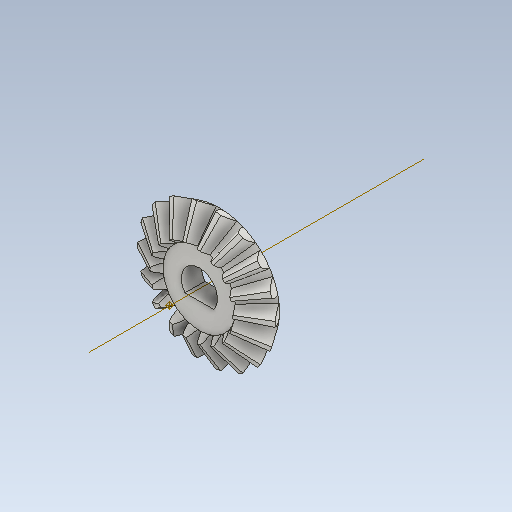
# Autodesk Inventor part: Коническая зубчатая передача2
Saved by Autodesk Inventor 2020 (Build 240168000, 168)
## iProperties
Created: 2021-02-28
Part Number: Коническая зубчатая передача2
Material: Steel, Mild
Document SubType Name: Modeling
Designer: Антон
Categories: <?xml version="1.0" encoding="UTF-16"?> <MemberInstance><Categories><FamilyTemplate><FamilyTemplateParameter ValueType="xs:double" Id="1" ObjectReferenceKey="da_z" ObjectType="kUserParameterObject"/><FamilyTemplateParameter ValueType="xs:double" Id="2" ObjectReferenceKey="da_b" ObjectType="kUserParameterObject"/><FamilyTemplateParameter ValueType="xs:double" Id="3" ObjectReferenceKey="da_beta" ObjectType="kUserParameterObject"/><FamilyTemplateParameter ValueType="xs:double" Id="4" ObjectReferenceKey="da_dae" ObjectType="kUserParameterObject"/><FamilyTemplateParameter ValueType="xs:double" Id="5" ObjectReferenceKey="da_ve" ObjectType="kUserParameterObject"/><FamilyTemplateParameter ValueType="xs:double" Id="6" ObjectReferenceKey="da_omega" ObjectType="kUserParameterObject"/><FamilyTemplateParameter ValueType="xs:string" Id="7" ObjectReferenceKey="EAIAABAAAAAAHwAAAAAAAIAAAAAAAAAA" ObjectType="83914240" SubObjectId="SurfaceGeometry"/></FamilyTemplate><ParamToTemplateMap><ParamToTemplate CategoryParameter="//CategoryParameter[@InternalName='046C89C9-8512-4d59-83FE-43B91F4F132A']" TemplateParameter="1"/><ParamToTemplate CategoryParameter="//CategoryParameter[@InternalName='2552DF32-E462-4b46-AEBF-C6C7768E72AC']" TemplateParameter="2"/><ParamToTemplate CategoryParameter="//CategoryParameter[@InternalName='C9EE641D-15FC-4fae-A226-E94C4372FDD7']" TemplateParameter="3"/><ParamToTemplate><ParamToTemplate CategoryParameter="//CategoryParameter[@InternalName='00B6519A-459B-49c7-AD84-2E56D39A5744']" ConstantValue="-0.000000"/></ParamToTemplate><ParamToTemplate><ParamToTemplate CategoryParameter="//CategoryParameter[@InternalName='04B31F0E-C7A6-4894-AA32-9629BEFACF47']" ConstantValue="1.000000"/></ParamToTemplate><ParamToTemplate><ParamToTemplate CategoryParameter="//CategoryParameter[@InternalName='43CBEC2E-7847-49e7-A936-2F7889FCB2D9']" ConstantValue="0.200000"/></ParamToTemplate><ParamToTemplate><ParamToTemplate CategoryParameter="//CategoryParameter[@InternalName='B1EFC894-105D-4ebd-86BF-FA20ED196853']" ConstantValue="0.300000"/></ParamToTemplate><ParamToTemplate><ParamToTemplate CategoryParameter="//CategoryParameter[@InternalName='51175063-3D10-4879-93E8-6246FE8B403D']" ConstantValue="2060000000.000000"/></ParamToTemplate><ParamToTemplate><ParamToTemplate CategoryParameter="//CategoryParameter[@InternalName='A3A52E27-4454-46a9-B0BD-C932399B70AF']" ConstantValue="0.300000"/></ParamToTemplate><ParamToTemplate CategoryParameter="//CategoryParameter[@InternalName='2A200944-5A8C-41ca-B96E-8520D2E510F1']" TemplateParameter="4"/><ParamToTemplate><ParamToTemplate CategoryParameter="//CategoryParameter[@InternalName='1A637F62-92C8-44bc-B81F-10802510B579']" ConstantValue="1.151274"/></ParamToTemplate><ParamToTemplate CategoryParameter="//CategoryParameter[@InternalName='B52DD4BE-6863-48fb-BF58-89EF6F9EC65C']" TemplateParameter="5"/><ParamToTemplate><ParamToTemplate CategoryParameter="//CategoryParameter[@InternalName='3956BFF2-84D2-457d-93C2-9B0613DEBA67']" ConstantValue="0.311351"/></ParamToTemplate><ParamToTemplate CategoryParameter="//CategoryParameter[@InternalName='739CFA02-461B-4bf8-8049-181FCAD8B28F']" TemplateParameter="6"/><ParamToTemplate><ParamToTemplate CategoryParameter="//CategoryParameter[@InternalName='A27E999F-E2CE-4481-8A2A-EBF499C4C3C5']" ConstantValue="-0.000000"/></ParamToTemplate><ParamToTemplate><ParamToTemplate CategoryParameter="//CategoryParameter[@InternalName='9E1B4470-B2D3-4ff1-B813-535BB4CDF51A']" ConstantValue="3520000.000000"/></ParamToTemplate><ParamToTemplate><ParamToTemplate CategoryParameter="//CategoryParameter[@InternalName='F8452263-BFF6-458c-9FB1-07C4B99E95CD']" ConstantValue="11400000.000000"/></ParamToTemplate><ParamToTemplate><ParamToTemplate CategoryParameter="//CategoryParameter[@InternalName='3E3BB259-FD49-497f-8171-6EBC954A3479']" ConstantValue="2.000000"/></ParamToTemplate><ParamToTemplate CategoryParameter="//CategoryParameter[@InternalName='27C3BAF2-7550-4e4b-AE2C-0DB134B7D9B7']" TemplateParameter="7"/></ParamToTemplateMap><Category DisplayName="Gear" InternalName="DC85795E-93AB-48d5-8EEE-5A27447B64BD" Mnemonic="Gear"><CategoryParameter DisplayName="z" InternalName="046C89C9-8512-4d59-83FE-43B91F4F132A" Mnemonic="z"/><CategoryParameter DisplayName="b" InternalName="2552DF32-E462-4b46-AEBF-C6C7768E72AC" Mnemonic="b"/><CategoryParameter DisplayName="||b|" InternalName="C9EE641D-15FC-4fae-A226-E94C4372FDD7" Mnemonic="beta"/><CategoryParameter DisplayName="x" InternalName="00B6519A-459B-49c7-AD84-2E56D39A5744" Mnemonic="x"/><CategoryParameter DisplayName="a*" InternalName="04B31F0E-C7A6-4894-AA32-9629BEFACF47" Mnemonic="a"/><CategoryParameter DisplayName="c*" InternalName="43CBEC2E-7847-49e7-A936-2F7889FCB2D9" Mnemonic="c"/><CategoryParameter DisplayName="r|.f|*" InternalName="B1EFC894-105D-4ebd-86BF-FA20ED196853" Mnemonic="rf"/><CategoryParameter DisplayName="E" InternalName="51175063-3D10-4879-93E8-6246FE8B403D" Mnemonic="E"/><CategoryParameter DisplayName="||m|" InternalName="A3A52E27-4454-46a9-B0BD-C932399B70AF" Mnemonic="mi"/><Category DisplayName="BevelGear" InternalName="0C98F69A-0C2B-4791-B2FE-7691BB227E77" Mnemonic="BevelGear"><CategoryParameter DisplayName="d|.ae|" InternalName="2A200944-5A8C-41ca-B96E-8520D2E510F1" Mnemonic="dae"/><CategoryParameter DisplayName="d|.ai|" InternalName="1A637F62-92C8-44bc-B81F-10802510B579" Mnemonic="dai"/><CategoryParameter DisplayName="J|.e|" InternalName="B52DD4BE-6863-48fb-BF58-89EF6F9EC65C" Mnemonic="ve"/><CategoryParameter DisplayName="J|.i|" InternalName="3956BFF2-84D2-457d-93C2-9B0613DEBA67" Mnemonic="vi"/><CategoryParameter DisplayName="||S|" InternalName="739CFA02-461B-4bf8-8049-181FCAD8B28F" Mnemonic="omega"/><CategoryParameter DisplayName="x|.t|" InternalName="A27E999F-E2CE-4481-8A2A-EBF499C4C3C5" Mnemonic="xt"/><CategoryParameter DisplayName="||s||.Flim|" InternalName="9E1B4470-B2D3-4ff1-B813-535BB4CDF51A" Mnemonic="sFlim"/><CategoryParameter DisplayName="||s||.Hlim|" InternalName="F8452263-BFF6-458c-9FB1-07C4B99E95CD" Mnemonic="sHlim"/><CategoryParameter DisplayName="тип" InternalName="3E3BB259-FD49-497f-8171-6EBC954A3479" Mnemonic="type"/><CategoryParameter DisplayName="PitchDiameter" InternalName="27C3BAF2-7550-4e4b-AE2C-0DB134B7D9B7" Mnemonic="IDS_PITCHDIAM"/></Category></Category></Categories></MemberInstance>
Mass: 60.9118 g
Surface Area: 34.3074 cm^2
Volume: 7.7496 cm^3
Density: 7.86 g/cm^3
Appearance: Steel
CustomPartVersion: 1
Author: Антон
Autodesk Inventor part; units mm, degrees
ref_plane "Плоскость сетки 2" through (0, 0, 0) normal (0.9848078, 0.1736482, 0) x (0, 0, 1)
sketch "Эскиз тела зубьев" plane through (0, 0, 0) normal (1, 0, 0) x (0, 1, 0)
  line L0 (0, 0) -> (8.33436, -6.99846) construction
  line L1 (8.33436, -6.99846) -> (9.5547, -5.16795)
  line L2 (9.5547, -5.16795) -> (0, 0) construction
  line L3 (9, -6) -> (0, 0) construction
  line L4 (5.021159, -4.216326) -> (5.756371, -3.113508)
  line L5 (8.33436, -6.99846) -> (5.021159, -4.216326)
  line L6 (9.5547, -5.16795) -> (5.756371, -3.113508)
  line L7 (0, -8.398152) -> (0, 1.399692)
  line L8 (0, -6) -> (9.5547, -6) construction
  dimension "d0" = 18
  dimension "d1" = 16.66872
  dimension "d2" = 19.1094
  dimension "d3" = 4.3
  dimension "d4" = 5.16795
  constraints: 16 end point, 4 point on line, 3 perpendicular, 2 collinear, 1 horizontal alignment, 1 vertical alignment
  measures "d0" diameter of L3.start L7
  measures "d1" diameter of L0.end L7
  measures "d2" diameter of L1.end L7
  measures "d3" distance between parallel lines of L1 L4
  measures "d4" vertical distance of L1.end L0.start
revolve "Тело зубьев" add sketch "Эскиз тела зубьев" angle 360 about axis through (0, 0, 0) along (0, 0, 1)
ref_plane "Плоскость зуба" through (0, 9, -6) normal (0, -0.8320503, 0.5547002) x (1, 0, 0)
sketch "Создать эскиз" plane through (0, 9, -6) normal (0, -0.8320503, 0.5547002) x (1, 0, 0)
  line L0 (0, -19.804283) -> (0, 5.250835)
  arc A0 (-0.390052, -1.464) -> (-1.790678, 1.570131) centre (-6.219235, -2.31454) ccw
  arc A1 (1.790678, 1.570131) -> (0.390052, -1.464) centre (6.219235, -2.31454) ccw
  line L1 (-0.390052, -1.464) -> (0.390052, -1.464)
  arc A2 (1.790678, 1.570131) -> (-1.790678, 1.570131) centre (0, -16.22498) ccw
  dimension "d7" = 5.89091
  dimension "d8" = 6.21924
  dimension "d9" = 13.91044
  dimension "d57" = 17.88498
  dimension "d58" = 14.76098
  constraints: 6 point on circle, 3 centre point, 3 symmetric about line, 2 end point, 1 coincident, 1 perpendicular, 1 other
  measures "d7" radius of A0
  measures "d8" horizontal distance of point (0, -16.225) A0.centre
  measures "d9" vertical distance of point (0, -16.225) A0.centre
  measures "d57" radius of A2
  measures "d58" distance from line of A2.centre L1
ref_plane "Конечная плоскость" through (0, 5.330658, -3.553772) normal (0, -0.8320503, 0.5547002) x (1, 0, 0)
sketch "Конечный эскиз" plane through (0, 5.330658, -3.553772) normal (0, -0.8320503, 0.5547002) x (1, 0, 0)
  line L0 (0, -15.025617) -> (0, 3.983837)
  arc A0 (-0.231026, -0.86712) -> (-1.06061, 0.929981) centre (-3.683624, -1.370892) ccw
  arc A1 (1.06061, 0.929981) -> (0.231026, -0.86712) centre (3.683624, -1.370892) ccw
  line L1 (-0.231026, -0.86712) -> (0.231026, -0.86712)
  arc A2 (1.06061, 0.929981) -> (-1.06061, 0.929981) centre (0, -9.609981) ccw
  dimension "d12" = 3.48916
  dimension "d15" = 3.68362
  dimension "d16" = 8.23909
  dimension "d59" = 10.59319
  dimension "d60" = 8.74286
  constraints: 6 point on circle, 3 centre point, 3 symmetric about line, 2 end point, 1 coincident, 1 other
  measures "d12" radius of A0
  measures "d15" horizontal distance of A0.centre point (0, -9.61)
  measures "d16" vertical distance of A0.centre point (0, -9.61)
  measures "d59" radius of A2
  measures "d60" distance from line of A2.centre L1
loft "Loft" cut profiles "Создать эскиз", "Конечный эскиз"
pattern_circular "Circular Pattern" count 18 over 360 about axis through (0, 0, 0) along (0, 0, 1) of "Loft"
sketch3d "3D эскиз: справа"
ref_plane "Конечная плоскость: справа" through (-1.067649, 5.222647, -3.553772) normal (0.1666469, -0.8151911, 0.5547002) x (0.9797378, 0.2002846, 0)
sketch "Конечный эскиз: справа" plane through (-1.067649, 5.222647, -3.553772) normal (0.1666469, -0.8151911, 0.5547002) x (0.9797378, 0.2002846, 0)
  arc A0 (-0.231026, -0.86712) -> (-1.06061, 0.929981) centre (-3.683624, -1.370892) ccw
  line L0 (0, -16.4637) -> (0, 5.42192)
  arc A1 (1.06061, 0.929981) -> (0.231026, -0.86712) centre (3.683624, -1.370892) ccw
  line L1 (-0.231026, -0.86712) -> (0.231026, -0.86712)
  arc A2 (1.06061, 0.929981) -> (-1.06061, 0.929981) centre (0, -9.609981) ccw
  dimension "d70" = 3.68362
  dimension "d71" = 8.23909
  dimension "d72" = 3.48916
  dimension "d73" = 8.74286
  dimension "d74" = 10.59319
  constraints: 6 point on circle, 3 centre point, 3 symmetric about line, 2 end point, 1 coincident, 1 perpendicular, 1 other
  measures "d70" horizontal distance of A2.centre A0.centre
  measures "d71" vertical distance of point (0, -9.61) A0.centre
  measures "d72" radius of A0
  measures "d73" distance from line of point (0, -9.61) L1
  measures "d74" radius of A2
feature "Лофт: справа" [suppressed]
pattern_circular "Круговой массив: справа" [suppressed]
sketch3d "3D эскиз: слева"
ref_plane "Конечная плоскость: cлева" through (1.05823, 5.222647, -3.549683) normal (-0.1652755, -0.8156788, 0.5543934) x (0.9800831, -0.1985877, 0)
sketch "Конечный эскиз: слева" plane through (1.05823, 5.222647, -3.549683) normal (-0.1652755, -0.8156788, 0.5543934) x (0.9800831, -0.1985877, 0)
  line L0 (0, -17.235664) -> (0, 6.212881)
  arc A0 (-0.231026, -0.869482) -> (-1.06061, 0.92762) centre (-3.683624, -1.373253) ccw
  arc A1 (1.06061, 0.92762) -> (0.231026, -0.869482) centre (3.683624, -1.373253) ccw
  line L1 (-0.231026, -0.869482) -> (0.231026, -0.869482)
  ellipse E0 centre (0, -2.591232) end of major axis (5.756371, -2.591232) minor radius 3.191294
  arc A2 (1.06061, 0.92762) -> (-1.06061, 0.92762) centre (0, -9.612342) ccw
  dimension "d56" = 3.19129
  dimension "d30" = 3.48916
  dimension "d31" = 3.68362
  dimension "d32" = 8.23909
  dimension "d61" = 10.59319
  dimension "d62" = 8.74286
  constraints: 6 point on circle, 3 centre point, 3 symmetric about line, 2 end point, 1 coincident, 2 other
  measures "d30" radius of A0
  measures "d31" horizontal distance of point (0, -9.612) A0.centre
  measures "d32" vertical distance of A0.centre point (0, -9.612)
  measures "d61" radius of A2
  measures "d62" distance from line of point (0, -9.612) L1
feature "Лофт: слева" [suppressed]
pattern_circular "Круговой массив: слева" [suppressed]
sketch "Эскиз тела" plane through (0, 0, 0) normal (1, 0, 0) x (0, 1, 0)
  line L0 (0, -7.321964) -> (0, -5.057437)
  line L1 (8.33436, -6.99846) -> (5.021159, -4.216326)
  line L2 (5.021159, -4.216326) -> (0, -4.216326)
  line L3 (8.33436, -6.99846) -> (0, -6.99846)
  constraints: 4 end point, 2 perpendicular, 2 point on line
sketch "Эскиз тела outline for Фиксировать тело" plane through (0, 0, 0) normal (1, 0, 0) x (0, 1, 0)
  line L0 (0, -6.99846) -> (8.33436, -6.99846)
  line L1 (0, -4.216326) -> (0, -6.99846)
  line L2 (5.021159, -4.216326) -> (0, -4.216326)
  line L3 (8.33436, -6.99846) -> (5.021159, -4.216326)
revolve "Фиксировать тело" add sketch "Эскиз тела outline for Фиксировать тело" angle 360 about axis through (0, 0, 0) along (0, 0, 1)
sketch "Sketch6" plane through (0, 0, 0) normal (1, 0, 0) x (0, 1, 0)
  line L0 (9, -6) -> (0, 0) projected
  line L1 (0, -7.2) -> (0, 1.2) projected
surface revolve "Средний диаметр" sketch "Sketch6" angle 360 about axis through (0, 0, 0) along (0, 0, 1) shown no curves L0
sketch "Эскиз8" plane through (0, 0, -4.216326) normal (0, 0, 1) x (1, 0, 0)
  circle A0 centre (0, 0) radius 2.5
  line L0 (2.5, -1.5) -> (-2.5, -1.5)
  line L1 (-2.5, -1.5) -> (-2.5, 1.5)
  line L2 (-2.5, 1.5) -> (2.5, 1.5)
  line L3 (2.5, 1.5) -> (2.5, -1.5)
  line L4 (2.5, -1.5) -> (-2.5, 1.5) construction
  line L5 (-2.5, -1.5) -> (2.5, 1.5) construction
  point P0 (-2, -1.5)
  point P1 (2, -1.5)
  dimension "d103" = 5
  dimension "d104" = 5
  dimension "d105" = 3
  constraints: 12 end point, 2 midpoint, 2 parallel, 1 centre point, 1 coincident, 1 horizontal, 1 perpendicular
  measures "d103" diameter of A0
  measures "d104" distance of L1.end L2.end
  measures "d105" distance of L0.end L1.end
extrude "Выдавливание1" cut sketch "Эскиз8" against normal through all contours A0 L0 L2 | L2 A0
equation "\"d0\" = da_de"
equation "\"d1\" = da_dfe"
equation "\"d2\" = da_dae"
equation "\"d3\" = da_b"
equation "\"d4\" = da_ve"
equation "\"d7\" = fd_rr"
equation "\"d8\" = fd_x"
equation "\"d9\" = fd_y"
equation "\"d57\" = 0.5 * fd_dva + 0.3 * da_he"
equation "\"d58\" = 0.5 * fd_dva - 1.12 * da_he"
equation "\"da_teethtype\" = 0"
equation "\"da_b\" = 4.3"
equation "\"da_de\" = 18"
equation "\"da_dae\" = 19.1094"
equation "\"da_dfe\" = 16.66872"
equation "\"da_le\" = 10.81665"
equation "\"da_omega\" = 90deg"
equation "\"da_beta\" = 0"
equation "\"da_delta\" = 56.309932deg"
equation "\"da_alpha\" = 20deg"
equation "\"da_he\" = 2.2"
equation "\"da_ve\" = 5.16795"
equation "\"da_zv\" = 32.449961"
equation "\"fd_loft\" = da_b + 0.05 * da_he"
equation "\"fd_x\" = fd_x1 + fd_x2"
equation "\"fd_y\" = fd_y1 - fd_y2"
equation "\"fd_dd\" = fd_dva - 0.8 * da_he"
equation "\"da_dvw\" = 32.44996"
equation "\"d11\" = fd_loft"
equation "\"da_dm\" = 14.42218"
equation "\"da_x\" = 0"
equation "\"da_m\" = 1"
equation "\"d50\" = da_omega"
equation "\"fd_rr\" = 5.890908"
equation "\"fd_dva\" = 34.449961"
equation "\"fd_x1\" = 0.793808"
equation "\"fd_x2\" = 5.425428"
equation "\"fd_y1\" = 16.205551"
equation "\"fd_y2\" = 2.29511"
body "Solid1"
body "Srf1"
